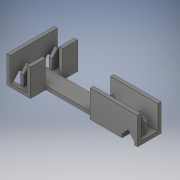
# Autodesk Inventor part: IPC_35
Saved by Autodesk Inventor 2019 (Build 230136000, 136)
## iProperties
Created: 2021-08-31
Part Number: IPC_35
Material: Generic
Document SubType Name: Modeling
Designer: zachm
Density: 1 g/cm^3
Appearance: Anodized - Light Gray
Author: zachm
Autodesk Inventor part; units mm, degrees
ref_plane "YZ Plane" through (0, 0, 0) normal (1, 0, 0) x (0, 1, 0)
ref_plane "XZ Plane" through (0, 0, 0) normal (0, 1, 0) x (-1, 0, 0)
sketch "Sketch1" plane through (0, 0, 0) normal (0, 1, 0) x (-1, 0, 0)
  line L0 (0, 0) -> (-5, 0)
  line L1 (-5, 0) -> (-5, -10)
  line L2 (-5, -10) -> (0, -10)
  line L3 (0, -10) -> (0, 0)
  line L4 (-15, -2.5) -> (-25, -2.5)
  line L5 (-25, -2.5) -> (-25, -7.5)
  line L6 (-25, -7.5) -> (-15, -7.5)
  line L7 (-15, -7.5) -> (-15, -2.5)
  line L8 (-5, -3.25) -> (-15, -3.25)
  line L9 (-15, -3.25) -> (-15, -6.75)
  line L10 (-15, -6.75) -> (-5, -6.75)
  line L11 (-5, -6.75) -> (-5, -3.25)
  dimension "d0" = 5
  dimension "d1" = 10
  dimension "d2" = 10
  dimension "d3" = 5
  dimension "d4" = 10
  dimension "d5" = 3.25
  dimension "d6" = 3.25
  dimension "d7" = 0.75
  constraints: 24 end point, 6 parallel, 3 horizontal, 3 perpendicular, 2 point on line
  measures "d0" distance of L2.end L1.end
  measures "d1" distance of L1.end L0.end
  measures "d2" distance of L6.end L5.end
  measures "d3" distance of L5.end L4.end
  measures "d4" distance of L9.end L10.end
  measures "d5" distance between parallel lines of L0 L8
  measures "d6" distance between parallel lines of L2 L10
  measures "d7" distance between parallel lines of L6 L10
extrude "Extrusion1" add sketch "Sketch1" along normal blind 0.75
sketch "Sketch2" plane through (0, 0.75, 0) normal (0, 1, 0) x (1, 0, 0)
  line L0 (15, 2.5) -> (25, 2.5) projected
  line L1 (25, 2.5) -> (25, 7.5) projected
  line L2 (15, 2.5) -> (25, 2.5)
  line L3 (25, 2.5) -> (25, 3.25)
  line L4 (25, 3.25) -> (15, 3.25)
  line L5 (15, 3.25) -> (15, 2.5)
  line L6 (15, 7.5) -> (15, 6.75) projected
  line L7 (15, 6.75) -> (25, 6.75)
  line L8 (25, 6.75) -> (25, 7.5)
  line L9 (25, 7.5) -> (15, 7.5)
  line L10 (15, 7.5) -> (15, 6.75)
  line L11 (0, 0) -> (5, 0) projected
  line L12 (5, 10) -> (0, 10) projected
  line L13 (0, 0) -> (0.75, 0)
  line L14 (0.75, 0) -> (0.75, 10)
  line L15 (0.75, 10) -> (0, 10)
  line L16 (0, 10) -> (0, 0)
  line L17 (5, 0) -> (4.25, 0)
  line L18 (4.25, 10) -> (5, 10)
  line L19 (5, 3.25) -> (4.25, 3.25)
  line L20 (4.25, 6.75) -> (5, 6.75)
  line L21 (5, 10) -> (5, 6.75)
  line L22 (5, 3.25) -> (5, 0)
  line L23 (4.25, 0) -> (4.25, 3.25)
  line L24 (4.25, 6.75) -> (4.25, 10)
  dimension "d15" = 0.75
  dimension "d16" = 0.75
  dimension "d17" = 0.75
  dimension "d18" = 20
  dimension "d19" = 20.75
  dimension "d20" = 4.25
  dimension "d21" = 0.75
  constraints: 40 end point, 12 parallel, 5 horizontal, 5 perpendicular, 3 point on line
  measures "d15" distance of L3.end L2.end
  measures "d16" distance of L15.end L14.end
  measures "d17" distance of L18.start L18.end
  measures "d18" distance between parallel lines of L1 L21
  measures "d19" distance between parallel lines of L1 L23
  measures "d20" distance between parallel lines of L0 L20
  measures "d21" distance between parallel lines of L0 L19
extrude "Extrusion2" add sketch "Sketch2" along normal blind 5
sketch "Sketch6" plane through (0, 0.75, 0) normal (0, 1, 0) x (1, 0, 0)
  line L0 (0.75, 10) -> (0.75, 0) projected
  line L1 (4.25, 10) -> (0.75, 10) projected
  line L2 (0.75, 0) -> (4.25, 0) projected
  line L3 (2.125, 9.25) -> (2.875, 9.25)
  line L4 (2.875, 9.25) -> (2.875, 6.75)
  line L5 (2.875, 6.75) -> (2.125, 6.75)
  line L6 (2.125, 6.75) -> (2.125, 9.25)
  line L7 (2.125, 3.25) -> (2.875, 3.25)
  line L8 (2.875, 3.25) -> (2.875, 0.75)
  line L9 (2.875, 0.75) -> (2.125, 0.75)
  line L10 (2.125, 0.75) -> (2.125, 3.25)
  point P0 (0, 0)
  dimension "d55" = 0.75
  dimension "d56" = 0.75
  dimension "d57" = 2.5
  dimension "d58" = 2.5
  dimension "d59" = 0.75
  dimension "d60" = 0.75
  dimension "d61" = 1.375
  dimension "d62" = 1.375
  constraints: 16 end point, 4 parallel, 2 horizontal, 2 perpendicular
  measures "d55" distance between parallel lines of L4 L6
  measures "d56" distance between parallel lines of L8 L10
  measures "d57" distance of L3.end L4.end
  measures "d58" distance of L7.end L8.end
  measures "d59" distance between parallel lines of L1 L3
  measures "d60" distance between parallel lines of L2 L9
  measures "d61" distance between parallel lines of L0 L6
  measures "d62" distance between parallel lines of L0 L10
extrude "Extrusion7" add sketch "Sketch6" along normal blind 3.5
sketch "Sketch7" plane through (0, 0.75, 0) normal (0, 1, 0) x (1, 0, 0)
  line L0 (2.875, 9.25) -> (2.875, 6.75) projected
  line L1 (2.875, 6.75) -> (2.125, 6.75) projected
  line L2 (2.125, 6.75) -> (2.125, 9.25) projected
  line L3 (2.125, 9.25) -> (2.875, 9.25) projected
  line L4 (2.875, 3.25) -> (2.875, 0.75) projected
  line L5 (2.875, 0.75) -> (2.125, 0.75) projected
  line L6 (2.125, 0.75) -> (2.125, 3.25) projected
  line L7 (2.125, 3.25) -> (2.875, 3.25) projected
  line L8 (15, 3.25) -> (25, 3.25) projected
  line L9 (25, 3.25) -> (25, 6.75) projected
  line L10 (25, 6.75) -> (15, 6.75) projected
  line L11 (15, 6.75) -> (5, 6.75) projected
  line L12 (5, 6.75) -> (4.25, 6.75) projected
  line L13 (4.25, 6.75) -> (4.25, 10) projected
  line L14 (4.25, 10) -> (0.75, 10) projected
  line L15 (0.75, 10) -> (0.75, 0) projected
  line L16 (0.75, 0) -> (4.25, 0) projected
  line L17 (4.25, 0) -> (4.25, 3.25) projected
  line L18 (4.25, 3.25) -> (5, 3.25) projected
  line L19 (5, 3.25) -> (15, 3.25) projected
  line L20 (2.125, 3.25) -> (0.75, 3.25)
  line L21 (0.75, 3.25) -> (0.75, 0.75)
  line L22 (0.75, 0.75) -> (2.125, 0.75)
  line L23 (2.125, 0.75) -> (2.125, 3.25)
  line L24 (0.75, 10) -> (0.75, 0) projected
  line L25 (2.125, 6.75) -> (0.75, 6.75)
  line L26 (0.75, 6.75) -> (0.75, 9.25)
  line L27 (0.75, 9.25) -> (2.125, 9.25)
  line L28 (2.125, 9.25) -> (2.125, 6.75)
  point P0 (0, 0)
  dimension "d65" = 2.5
  dimension "d66" = 6
  constraints: 16 end point, 4 parallel, 2 horizontal, 2 perpendicular, 2 point on line
  measures "d65" distance between parallel lines of L1 L27
  measures "d66" distance between parallel lines of L1 L22
extrude "Extrusion8" cut sketch "Sketch7" against normal blind 0.75 contours L2 L25 L15 L27 | L20 L6 L22 L15
sketch "Sketch8" plane through (0, 0, -10) normal (-1, 0, 0) x (0, 0, 1)
  line L0 (0, 0) -> (10, 0) projected
  line L1 (9.25, 0) -> (6.75, 0)
  line L2 (8, 0) -> (8, 2.125) construction
  line L3 (6.75, 0) -> (6.75, 0.75)
  line L4 (6.75, 0) -> (7.5, 0) construction
  line L5 (9.25, 0) -> (9.25, 0.75)
  line L6 (9.25, 0) -> (10, 0) construction
  line L7 (9.25, 0.75) -> (8, 2.125)
  line L8 (6.75, 0.75) -> (8, 2.125)
  dimension "d69" = 2.5
  dimension "d70" = 0.75
  dimension "d71" = 2.125
  dimension "d72" = 0.75
  dimension "d73" = 90
  dimension "d74" = 0.75
  dimension "d75" = 90
  constraints: 16 end point, 4 perpendicular, 2 horizontal, 2 point on line, 1 midpoint, 1 vertical
  measures "d69" distance of L1.start L1.end
  measures "d70" distance of L0.end L1.start
  measures "d71" distance of L2.start L2.end
  measures "d72" distance of L1.end L3.end
  measures "d73" angle of L4 L3
  measures "d74" distance of L1.start L5.end
  measures "d75" angle of L6 L5
extrude "Extrusion9" cut sketch "Sketch8" against normal blind 0.75
sketch "Sketch9" plane through (2.125, 4.25, -3.25) normal (-1, 0, 0) x (0, 0, 1)
  line L0 (2.5, -3.5) -> (2.5, 0) projected
  line L1 (0, 0) -> (2.5, 0) projected
  line L2 (0, -3.5) -> (0, 0) projected
  line L3 (0, -3.5) -> (0, -4.25) projected
  line L4 (2.5, -4.25) -> (0, -4.25) projected
  line L5 (2.5, -3.5) -> (2.5, -4.25) projected
  line L6 (0, -3.5) -> (0, 0) projected
  line L7 (0, -1.375) -> (2.5, -1.375) construction
  line L8 (0, -1.375) -> (1.25, 0)
  line L9 (0, 0) -> (2.5, 0) projected
  line L10 (0, 0) -> (1.25, 0)
  line L11 (0, 0) -> (0, -1.375)
  line L12 (1.25, 0) -> (2.5, 0)
  line L13 (2.5, 0) -> (2.5, -1.375)
  line L14 (2.5, -1.375) -> (1.25, 0)
  point P0 (3.25, -4.25)
  dimension "d78" = 1.375
  constraints: 14 end point, 3 perpendicular, 2 collinear, 2 point on line, 1 midpoint
  measures "d78" distance between parallel lines of L1 L7
extrude "Extrusion10" cut sketch "Sketch9" against normal blind 0.75 contours L14 L1 L0 | L8 L2 L1
ref_plane "Work Plane1" through (0, 0, -5) normal (0, 0, 1) x (1, 0, 0)
mirror "Mirror1" about plane through (0, 0, -5) normal (0, 0, 1) of "Extrusion9", "Extrusion10"
sketch "Sketch10" plane through (15, 0, -2.5) normal (0, 0, 1) x (1, 0, 0)
  line L0 (10, 0) -> (0, 0) projected
  line L1 (9.25, 0) -> (6.75, 0)
  line L2 (10, 0) -> (10, 5.75) projected
  line L3 (6.75, 0) -> (6.75, 0.75)
  line L4 (10, 0.75) -> (0, 0.75) projected
  line L5 (9.25, 0) -> (9.25, 0.75)
  line L6 (8, 0) -> (8, 2.125) construction
  line L7 (8, 2.125) -> (6.75, 0.75)
  line L8 (8, 2.125) -> (9.25, 0.75)
  point P0 (-15, 0)
  dimension "d81" = 2.5
  dimension "d82" = 0.75
  dimension "d83" = 0.75
  dimension "d84" = 0.75
  dimension "d85" = 2.125
  constraints: 12 end point, 4 point on line, 1 midpoint, 1 perpendicular
  measures "d81" distance of L1.start L1.end
  measures "d82" distance from line of L2 L1.start
  measures "d83" distance of L1.end L3.end
  measures "d84" distance of L1.start L5.end
  measures "d85" distance of L6.start L6.end
extrude "Extrusion11" cut sketch "Sketch10" against normal blind 2.125 contours L0 L3 L4 L5 | L4 L7 L8
sketch "Sketch11" plane through (15, 0, -4.625) normal (0, 0, 1) x (1, 0, 0)
  line L0 (0, 0.75) -> (6.75, 0.75) projected
  line L1 (6.75, 0.75) -> (6.75, 2.875)
  line L2 (6.75, 2.875) -> (9.25, 2.875) construction
  line L3 (9.25, 2.875) -> (9.25, 0.75)
  line L4 (9.25, 0.75) -> (6.75, 0.75)
  line L5 (8, 2.875) -> (8, 4.25) construction
  line L6 (6.75, 2.875) -> (8, 4.25)
  line L7 (8, 4.25) -> (9.25, 2.875)
  point P0 (-15, 0)
  dimension "d88" = 2.125
  dimension "d89" = 2.5
  dimension "d90" = 1.375
  constraints: 14 end point, 3 perpendicular, 2 vertical, 1 midpoint
  measures "d88" distance of L0.end L1.end
  measures "d89" distance of L1.end L2.end
  measures "d90" distance of L5.start L5.end
extrude "Extrusion12" add sketch "Sketch11" against normal blind 0.75
sketch "Sketch12" plane through (0, 0.75, 0) normal (0, 1, 0) x (1, 0, 0)
  line L0 (15, 6.75) -> (5, 6.75) projected
  line L1 (15, 6.75) -> (20, 6.75) construction
  line L2 (25, 6.75) -> (15, 6.75) projected
  line L3 (20, 6.75) -> (20, 5) construction
  point P0 (0, 0)
  dimension "d93" = 5
  dimension "d94" = 1.75
  constraints: 4 end point, 1 midpoint, 1 perpendicular
  measures "d93" distance of L0.start L1.end
  measures "d94" distance of L1.end L3.end
pattern_circular "Circular Pattern2" count 2 over 360 about axis through (20, 0.75, -5) along (0, 1, 0) of "Extrusion12", "Extrusion11"
fillet "Fillet1" radius 0.05 43 edges at (0, 5.75, -5) (0.375, 5.75, 0) (0, 0, -0.375) (0, 0, -5) (0, 0, -9.625) (0, 2.875, 0) (20, 5.75, -7.5) (20, 5.75, -6.75) (15, 3.25, -6.75) (15, 5.75, -7.125) (25, 5.75, -7.125) (25, 3.25, -6.75) (15, 2.875, -7.5) (20, 5.75, -3.25) (15, 5.75, -2.875) (20, 5.75, -2.5) (15, 2.875, -2.5) (15, 3.25, -3.25) (25, 2.875, -2.5) (25, 3.25, -3.25) (25, 2.875, -7.5) (0.375, 5.75, -10) (0.75, 5.75, -5) (5, 5.75, -8.375) (4.25, 5.75, -8.375) (4.625, 5.75, -10) (4.625, 5.75, -6.75) (4.625, 5.75, -3.25) (5, 5.75, -1.625) (4.25, 5.75, -1.625) (4.625, 5.75, 0) (5, 2.875, 0) (4.25, 3.25, 0) (4.25, 3.25, -3.25) (4.25, 3.25, -6.75) (5, 3.25, -6.75) (5, 2.875, -10) (4.25, 3.25, -10) (5, 3.25, -3.25) (0.75, 3.25, -10) (0, 2.875, -10) (0.75, 3.25, 0) (22.375, 1.4375, -2.5)
fillet "Fillet1" radius 0.05 149 edges at (18.25, 2.875, -5) (18.25, 1.8125, -5.375) (18.25, 1.8125, -4.625) (15.75, 0.75, -6.0625) (18.25, 0.75, -6.0625) (25, 0.75, -5) (24.25, 0.75, -3.9375) (21.75, 0.75, -3.9375) (10, 0.75, -3.25) (2.5, 0.75, 0) (1.4375, 0.75, -0.75) (1.4375, 0.75, -3.25) (1.4375, 0.75, -6.75) (1.4375, 0.75, -9.25) (2.5, 0.75, -10) (10, 0.75, -6.75) (17, 4.25, -5) (17.625, 3.5625, -5.375) (17.625, 3.5625, -4.625) (17, 0, -5.375) (15.75, 1.8125, -5.375) (16.375, 3.5625, -5.375) (16.375, 3.5625, -4.625) (15.75, 1.8125, -4.625) (16.375, 1.4375, -6.75) (17.625, 1.4375, -6.75) (25, 3.25, -6.75) (20, 5.75, -6.75) (15, 3.25, -6.75) (15.75, 0, -6.4375) (15.75, 0.375, -7.5) (15.75, 2.875, -5) (18.25, 0, -6.4375) (18.25, 0.375, -7.5) (25, 2.875, -2.5) (25, 5.75, -2.875) (25, 3.25, -3.25) (25, 5.75, -7.125) (25, 2.875, -7.5) (25, 0, -5) (23.625, 1.4375, -3.25) (22.375, 1.4375, -3.25) (15, 3.25, -3.25) (20, 5.75, -3.25) (24.25, 0, -3.5625) (24.25, 0.375, -2.5) (24.25, 2.875, -5) (24.25, 1.8125, -4.625) (24.25, 1.8125, -5.375) (21.75, 1.8125, -5.375) (22.375, 3.5625, -5.375) (23.625, 3.5625, -5.375) (21.75, 2.875, -5) (21.75, 1.8125, -4.625) (21.75, 0, -3.5625) (21.75, 0.375, -2.5) (10, 0, -3.25) (5, 3.25, -3.25) (4.25, 3.25, -3.25) (4.625, 5.75, -3.25) (4.25, 3.25, 0) (4.25, 5.75, -1.625) (0, 2.875, 0) (0.375, 5.75, 0) (0.75, 3.25, 0) (4.625, 5.75, 0) (5, 2.875, 0) (2.5, 0, 0) (0.75, 3.25, -10) (0.75, 5.75, -5) (0.75, 1.4375, -1.375) (0.75, 1.4375, -2.625) (0.75, 1.4375, -7.375) (0.75, 1.4375, -8.625) (1.0625, 0, -0.75) (0, 0.375, -0.75) (2.125, 1.8125, -0.75) (2.5, 2.875, -0.75) (2.875, 1.8125, -0.75) (2.875, 3.5625, -1.375) (2.875, 3.5625, -2.625) (2.875, 1.8125, -3.25) (2.5, 2.875, -3.25) (2.125, 1.8125, -3.25) (1.0625, 0, -3.25) (0, 0.375, -3.25) (1.0625, 0, -6.75) (0, 0.375, -6.75) (2.125, 1.8125, -6.75) (2.5, 2.875, -6.75) (2.875, 1.8125, -6.75) (2.875, 3.5625, -7.375) (2.875, 3.5625, -8.625) (2.875, 1.8125, -9.25) (2.5, 2.875, -9.25) (2.125, 1.8125, -9.25) (1.0625, 0, -9.25) (0, 0.375, -9.25) (5, 2.875, -10) (4.625, 5.75, -10) (4.25, 3.25, -10) (0.375, 5.75, -10) (0, 2.875, -10) (2.5, 0, -10) (4.25, 3.25, -6.75) (4.25, 5.75, -8.375) (5, 3.25, -6.75) (4.625, 5.75, -6.75) (10, 0, -6.75) (16.375, 1.4375, -7.5) (17.625, 1.4375, -7.5) (15, 5.75, -7.125) (20, 5.75, -7.5) (15, 2.875, -7.5) (15, 0, -7.125) (24.625, 0, -2.5) (23, 0, -4.625) (18.375, 0, -2.5) (15, 0, -2.875) (5, 0, -1.625) (0, 0, -0.375) (2.125, 0, -2) (0, 0, -5) (2.125, 0, -8) (0, 0, -9.625) (5, 0, -8.375) (15.375, 0, -7.5) (21.625, 0, -7.5) (22.375, 1.4375, -2.5) (23.625, 1.4375, -2.5) (20, 5.75, -2.5) (15, 2.875, -2.5) (15, 5.75, -2.875) (23.625, 3.5625, -4.625) (22.375, 3.5625, -4.625) (23, 4.25, -5) (5, 5.75, -1.625) (0, 1.4375, -8.625) (0, 1.4375, -7.375) (0, 1.4375, -2.625) (0, 1.4375, -1.375) (0, 5.75, -5) (2.125, 3.5625, -1.375) (2.125, 3.5625, -2.625) (2.5, 4.25, -2) (2.125, 3.5625, -7.375) (2.125, 3.5625, -8.625) (2.5, 4.25, -8) (5, 5.75, -8.375)
fillet "Fillet1" radius 0.05 47 edges at (18.25, 0.75, -5) (15.375, 0.75, -6.75) (15.75, 0.75, -5) (17, 0.75, -4.625) (21.625, 0.75, -6.75) (24.625, 0.75, -3.25) (24.25, 0.75, -5) (23, 0.75, -5.375) (21.75, 0.75, -5) (18.375, 0.75, -3.25) (4.625, 0.75, -3.25) (4.25, 0.75, -1.625) (0.75, 0.75, -0.375) (2.5, 0.75, -0.75) (2.875, 0.75, -2) (2.5, 0.75, -3.25) (0.75, 0.75, -5) (2.5, 0.75, -6.75) (2.875, 0.75, -8) (2.5, 0.75, -9.25) (0.75, 0.75, -9.625) (4.25, 0.75, -8.375) (4.625, 0.75, -6.75) (18.25, 0.375, -5.375) (15.75, 0.375, -5.375) (15.75, 0.75, -7.125) (18.25, 0.75, -7.125) (24.25, 0.75, -2.875) (24.25, 0.375, -4.625) (21.75, 0.75, -2.875) (21.75, 0.375, -4.625) (5, 0.375, -3.25) (15, 0.375, -3.25) (2.125, 0.375, -0.75) (0.375, 0.75, -0.75) (2.125, 0.375, -3.25) (0.375, 0.75, -3.25) (0.375, 0.75, -6.75) (2.125, 0.375, -6.75) (2.125, 0.375, -9.25) (0.375, 0.75, -9.25) (15, 0.375, -6.75) (5, 0.375, -6.75) (17, 2.125, -7.125) (23, 2.125, -2.875) (0.375, 2.125, -2) (0.375, 2.125, -8)
body "Solid1"
